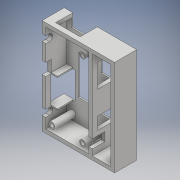
# Autodesk Inventor part: HousingTop
Saved by Autodesk Inventor 2017 (Build 210142000, 142)
## iProperties
Created: 2017-02-14
Part Number: HousingTop
Material: Generic
Document SubType Name: Modeling
Designer: William
Density: 1 g/cm^3
Appearance: Default
Author: William
Autodesk Inventor part; units mm, degrees
ref_plane "YZ Plane" through (0, 0, 0) normal (1, 0, 0) x (0, 1, 0)
ref_plane "XZ Plane" through (0, 0, 0) normal (0, 1, 0) x (-1, 0, 0)
ref_plane "XY Plane" through (0, 0, 0) normal (0, 0, 1) x (1, 0, 0)
sketch "Sketch1" plane through (0, 0, 0) normal (0, 1, 0) x (-1, 0, 0)
  circle A0 centre (0, 0) radius 1.6
  circle A1 centre (0, -62) radius 1.6
  circle A2 centre (25, -62) radius 1.6
  circle A3 centre (12, -31) radius 1.6
  circle A4 centre (12, -31) radius 2.5
  circle A5 centre (0, -62) radius 2.5
  circle A6 centre (25, -62) radius 2.5
  circle A7 centre (0, 0) radius 2.5
  line L0 (30, 5) -> (-5, 5)
  line L1 (-5, 5) -> (-5, -67)
  line L2 (-5, -67) -> (30, -67)
  line L3 (30, -67) -> (30, 5)
  line L4 (33, 8) -> (-8, 8)
  line L5 (-8, 8) -> (-8, -70)
  line L6 (-8, -70) -> (33, -70)
  line L7 (33, -70) -> (33, 8)
  dimension "d0" = 3.2
  dimension "d1" = 3.2
  dimension "d2" = 62
  dimension "d3" = 3.2
  dimension "d4" = 25
  dimension "d5" = 3.2
  dimension "d6" = 31
  dimension "d7" = 12
  dimension "d8" = 5
  dimension "d9" = 5
  dimension "d10" = 5
  dimension "d11" = 5
  dimension "d12" = 5
  dimension "d13" = 5
  dimension "d14" = 5
  dimension "d15" = 5
  dimension "d16" = 3
  dimension "d17" = 3
  dimension "d18" = 3
  dimension "d19" = 3
  dimension "d20" = 0
  constraints: 16 end point, 8 centre point, 5 coincident, 4 parallel, 2 horizontal, 2 perpendicular
  measures "d0" diameter of A0
  measures "d1" diameter of A1
  measures "d2" distance of point (0, 0) A1.centre
  measures "d3" diameter of A2
  measures "d4" distance of A1.centre A2.centre
  measures "d5" diameter of A3
  measures "d6" vertical distance of point (0, 0) A3.centre
  measures "d7" horizontal distance of point (0, 0) A3.centre
  measures "d8" diameter of A4
  measures "d9" diameter of A5
  measures "d10" diameter of A6
  measures "d11" diameter of A7
  measures "d12" distance from line of L2 A2.centre
  measures "d13" distance from line of A2.centre L3
  measures "d14" distance from line of L1 A0.centre
  measures "d15" distance from line of L0 point (0, 0)
  measures "d16" distance between parallel lines of L4 L0
  measures "d17" distance between parallel lines of L3 L7
  measures "d18" distance between parallel lines of L2 L6
  measures "d19" distance between parallel lines of L1 L5
  measures "d20" vertical distance of A1.centre A2.centre
extrude "Extrusion1" add sketch "Sketch1" along normal blind 17 contours A5 | A6 | A7 | L7 L6 L5 L4
sketch "Sketch2" plane through (0, 17, 0) normal (0, 1, 0) x (1, 0, 0)
  line L0 (-33, -8) -> (8, -8) projected
  line L1 (-33, 70) -> (-33, -8) projected
  line L2 (8, -8) -> (-33, -8)
  line L3 (-33, -8) -> (-33, 70)
  line L4 (-33, 70) -> (8, 70)
  line L5 (8, 70) -> (8, -8)
  point P0 (0, 0)
  constraints: 8 end point, 2 parallel, 1 horizontal, 1 perpendicular
extrude "Extrusion2" add sketch "Sketch2" along normal blind 2
sketch "Sketch3" plane through (0, 0, 0) normal (0, -1, 0) x (1, 0, 0)
  line L0 (-33, -70) -> (-33, 8) projected
  line L1 (-30, -67) -> (-30, 5) projected
  line L2 (-33, -30) -> (-30, -30)
  line L3 (-30, -30) -> (-30, -20)
  line L4 (-30, -20) -> (-33, -20)
  line L5 (-33, -20) -> (-33, -30)
  point P0 (0, 0)
  dimension "d25" = 20
  dimension "d26" = 10
  constraints: 8 end point, 2 parallel, 2 point on line, 1 horizontal, 1 perpendicular
  measures "d25" distance from line of point (0, 0) L4
  measures "d26" distance of L4.end L2.start
extrude "Extrusion3" cut sketch "Sketch3" against normal blind 4.5
sketch "Sketch4" plane through (0, 0, 0) normal (0, -1, 0) x (1, 0, 0)
  line L0 (-30, -6.75) -> (-33, -6.75)
  line L1 (-33, -6.75) -> (-33, -1.25)
  line L2 (-33, -1.25) -> (-30, -1.25)
  line L3 (-30, -1.25) -> (-30, -6.75)
  line L4 (-30, -6.75) -> (-33, -1.25) construction
  line L5 (-33, -6.75) -> (-30, -1.25) construction
  line L6 (-30, -20) -> (-30, 5) projected
  line L7 (-33, -20) -> (-33, 8) projected
  line L8 (-30, -58.75) -> (-33, -58.75)
  line L9 (-33, -58.75) -> (-33, -53.25)
  line L10 (-33, -53.25) -> (-30, -53.25)
  line L11 (-30, -53.25) -> (-30, -58.75)
  line L12 (-30, -58.75) -> (-33, -53.25) construction
  line L13 (-33, -58.75) -> (-30, -53.25) construction
  line L14 (-30, -67) -> (-30, -30) projected
  line L15 (-33, -70) -> (-33, -30) projected
  point P0 (0, 0)
  point P1 (-31.5, -4)
  point P2 (-31.5, -56)
  dimension "d29" = 0
  dimension "d30" = 5.5
  dimension "d31" = 0
  dimension "d32" = 4
  dimension "d33" = 0
  dimension "d34" = 0
  dimension "d35" = 56
  dimension "d36" = 5.5
  constraints: 24 end point, 4 midpoint, 4 parallel, 2 horizontal, 2 perpendicular
  measures "d29" distance between parallel lines of L6 L3
  measures "d30" distance of L0.end L1.end
  measures "d31" distance between parallel lines of L7 L1
  measures "d32" vertical distance of point (0, 0) point (-31.5, -4)
  measures "d33" distance between parallel lines of L14 L11
  measures "d34" distance between parallel lines of L15 L9
  measures "d35" vertical distance of point (0, 0) point (-31.5, -56)
  measures "d36" distance between parallel lines of L10 L8
extrude "Extrusion4" cut sketch "Sketch4" against normal blind 5.5
fillet "Fillet1" radius 2.5 4 edges at (-31.5, 5.5, -53.25) (-31.5, 5.5, -58.75) (-31.5, 5.5, -6.75) (-31.5, 5.5, -1.25)
sketch "Sketch5" plane through (0, 17, 0) normal (0, -1, 0) x (1, 0, 0)
  circle A0 centre (0, 0) radius 1.6 projected
  circle A1 centre (0, -62) radius 1.6 projected
  circle A2 centre (-25, -62) radius 1.6 projected
extrude "Extrusion5" cut sketch "Sketch5" against normal up to surface (2 mm away)
sketch "Sketch6" plane through (0, 19, 0) normal (0, 1, 0) x (1, 0, 0)
  line L0 (-23, 42.5) -> (-33, 42.5)
  line L1 (-33, 42.5) -> (-33, 52.5)
  line L2 (-33, 52.5) -> (-23, 52.5)
  line L3 (-23, 52.5) -> (-23, 42.5)
  line L4 (-23, 42.5) -> (-33, 52.5) construction
  line L5 (-33, 42.5) -> (-23, 52.5) construction
  line L6 (-33, -8) -> (-33, 70) projected
  line L7 (-33, 70) -> (8, 70) projected
  line L8 (8, 70) -> (8, -8) projected
  line L9 (8, -8) -> (-33, -8) projected
  circle A0 centre (-25, 62) radius 1.6 projected
  circle A1 centre (0, 62) radius 1.6 projected
  circle A2 centre (0, 0) radius 1.6 projected
  line L10 (-23, 42.5) -> (-33, 42.5)
  line L11 (-33, 42.5) -> (-33, 30.5)
  line L12 (-33, 30.5) -> (-23, 30.5)
  line L13 (-23, 30.5) -> (-23, 42.5)
  point P0 (-28, 47.5)
  dimension "d42" = 47.5
  dimension "d43" = 10
  dimension "d44" = 2
  dimension "d45" = 10
  dimension "d48" = 10
  dimension "d49" = 12
  constraints: 20 end point, 4 parallel, 2 horizontal, 2 midpoint, 2 perpendicular
  measures "d42" vertical distance of point (0, 0) point (-28, 47.5)
  measures "d43" distance of L1.end L2.end
  measures "d44" distance from line of A0.centre L3
  measures "d45" distance of L2.end L0.start
  measures "d48" distance of L12.end L11.end
  measures "d49" distance of L11.end L10.end
extrude "Extrusion6" cut sketch "Sketch6" against normal blind 15 contours L13 L12 L6 L0 | L0 L1 L2 L3
sketch "Sketch7" plane through (0, 17, 0) normal (0, -1, 0) x (1, 0, 0)
  line L0 (-33, -52.5) -> (-30, -52.5) projected
  line L1 (-30, -52.5) -> (-23, -52.5) projected
  line L2 (-23, -52.5) -> (-23, -30.5) projected
  line L3 (-23, -30.5) -> (-30, -30.5) projected
  line L4 (-30, -30.5) -> (-33, -30.5) projected
  line L5 (-33, -30.5) -> (-33, 8) projected
  line L6 (-33, 8) -> (8, 8) projected
  line L7 (8, 8) -> (8, -70) projected
  line L8 (8, -70) -> (-33, -70) projected
  line L9 (-33, -70) -> (-33, -52.5) projected
  line L10 (-30, -52.5) -> (-30, -67) projected
  line L11 (-30, -67) -> (5, -67) projected
  line L12 (5, -67) -> (5, 5) projected
  line L13 (5, 5) -> (-30, 5) projected
  line L14 (-30, 5) -> (-30, -30.5) projected
  circle A0 centre (-25, -62) radius 1.6 projected
  circle A1 centre (-25, -62) radius 2.5 projected
  circle A2 centre (0, -62) radius 1.6 projected
  circle A3 centre (0, -62) radius 2.5 projected
  circle A4 centre (0, 0) radius 1.6 projected
  circle A5 centre (0, 0) radius 2.5 projected
  line L15 (-30, -30.5) -> (-25, -30.5)
  line L16 (-25, -30.5) -> (-25, -29.5)
  line L17 (-25, -29.5) -> (-30, -29.5)
  line L18 (-30, -29.5) -> (-30, -30.5)
  line L19 (-30, -52.5) -> (-25, -52.5)
  line L20 (-25, -52.5) -> (-25, -53.5)
  line L21 (-25, -53.5) -> (-30, -53.5)
  line L22 (-30, -53.5) -> (-30, -52.5)
  dimension "d50" = 5
  dimension "d51" = 1
  dimension "d52" = 5
  dimension "d53" = 1
  constraints: 16 end point, 4 parallel, 2 horizontal, 2 perpendicular
  measures "d50" distance of L17.end L16.end
  measures "d51" distance of L16.end L15.end
  measures "d52" distance of L20.end L21.end
  measures "d53" distance of L19.end L20.end
extrude "Extrusion7" add sketch "Sketch7" along normal up to surface (12.5 mm away) contours L1 L20 L21 L10 | L3 L14 L17 L16
sketch "Sketch8" plane through (0, 19, 0) normal (0, 1, 0) x (1, 0, 0)
  circle A0 centre (0, 0) radius 1.6 construction
  line L0 (0, 0) -> (0, 32.2706) construction
  line L1 (0, 32.2706) -> (-4.4901, 32.2706) construction
  line L2 (-4.4901, 32.2706) -> (-6.7761, 32.2706) construction
  line L3 (-6.7761, 32.2706) -> (-20.4921, 32.2706) construction
  line L4 (-20.4921, 32.2706) -> (-20.4921, 16.2706) construction
  line L5 (-20.4921, 16.2706) -> (-6.7761, 16.2706)
  line L6 (-6.7761, 16.2706) -> (-6.7761, 48.2706)
  line L7 (-6.7761, 48.2706) -> (-20.4921, 48.2706)
  line L8 (-20.4921, 48.2706) -> (-20.4921, 16.2706)
  dimension "d56" = 2.286
  dimension "d57" = 13.716
  dimension "d58" = 16
  dimension "d59" = 32
  constraints: 18 end point, 3 horizontal, 2 parallel, 2 perpendicular, 2 vertical
  measures "d56" distance of L1.end L2.end
  measures "d57" distance of L2.end L3.end
  measures "d58" distance of L3.end L4.end
  measures "d59" distance of L6.end L5.end
extrude "Extrusion8" cut sketch "Sketch8" against normal up to next
sketch "Sketch9" plane through (0, 19, 0) normal (0, 1, 0) x (1, 0, 0)
  line L0 (-33, -8) -> (8, -8) projected
  line L1 (-6, -8) -> (-26, -8)
  line L2 (-26, -8) -> (-26, 2)
  line L3 (-26, 2) -> (-6, 2)
  line L4 (-6, 2) -> (-6, -8)
  line L5 (8, 3) -> (-2, 3)
  line L6 (-2, 3) -> (-2, 22)
  line L7 (-2, 22) -> (8, 22)
  line L8 (8, 22) -> (8, 3)
  line L9 (-2, 41) -> (8, 41)
  line L10 (8, 41) -> (8, 51)
  line L11 (8, 51) -> (-2, 51)
  line L12 (-2, 51) -> (-2, 41)
  line L13 (-2, 41) -> (8, 51) construction
  line L14 (8, 41) -> (-2, 51) construction
  line L15 (8, -8) -> (8, 70) projected
  point P0 (0, 0)
  point P1 (3, 46)
  dimension "d62" = 10
  dimension "d63" = 6
  dimension "d64" = 20
  dimension "d65" = 10
  dimension "d66" = 3
  dimension "d67" = 22
  dimension "d68" = 10
  dimension "d69" = 0
  dimension "d70" = 46
  dimension "d71" = 10
  constraints: 28 end point, 6 parallel, 3 horizontal, 3 perpendicular, 2 midpoint, 1 point on line
  measures "d62" distance of L1.end L2.end
  measures "d63" distance from line of point (0, 0) L4
  measures "d64" distance of L2.end L3.end
  measures "d65" distance of L6.end L7.end
  measures "d66" distance from line of point (0, 0) L5
  measures "d67" vertical distance of point (0, 0) L7.end
  measures "d68" distance between parallel lines of L15 L12
  measures "d69" distance between parallel lines of L15 L10
  measures "d70" vertical distance of point (0, 0) point (3, 46)
  measures "d71" distance of L11.end L9.start
extrude "Extrusion9" cut sketch "Sketch9" against normal blind 15
sketch "Sketch10" plane through (8, 0, 8) normal (1, 0, 0) x (0, 0, -1)
  line L0 (0, 19) -> (11, 19) projected
  line L1 (78, 0) -> (78, 19) projected
  line L2 (0, 19) -> (78, 19)
  line L3 (78, 19) -> (78, 0)
  line L4 (78, 0) -> (0, 0)
  line L5 (0, 0) -> (0, 19)
  point P0 (8, 0)
  constraints: 8 end point, 2 parallel, 1 horizontal, 1 perpendicular
extrude "Extrusion10" add sketch "Sketch10" along normal blind 18
sketch "Sketch11" plane through (0, 0, 0) normal (0, -1, 0) x (1, 0, 0)
  line L0 (23, -67) -> (8, -67)
  line L1 (8, -67) -> (8, 5)
  line L2 (8, 5) -> (23, 5)
  line L3 (23, 5) -> (23, -67)
  line L4 (-33, -70) -> (26, -70) projected
  line L5 (26, 8) -> (26, -70) projected
  line L6 (5, -67) -> (5, -51) projected
  line L7 (-33, 8) -> (26, 8) projected
  point P0 (0, 0)
  dimension "d76" = 3
  dimension "d77" = 3
  dimension "d78" = 3
  dimension "d79" = 3
  constraints: 8 end point, 2 parallel, 1 horizontal, 1 perpendicular
  measures "d76" distance between parallel lines of L4 L0
  measures "d77" distance between parallel lines of L5 L3
  measures "d78" distance between parallel lines of L6 L1
  measures "d79" distance between parallel lines of L7 L2
extrude "Extrusion11" cut sketch "Sketch11" against normal up to surface (17 mm away)
sketch "Sketch12" plane through (0, 0, 0) normal (0, -1, 0) x (1, 0, 0)
  line L0 (8, -51) -> (8, -67) projected
  line L1 (5, 5) -> (5, -67) projected
  line L2 (8, -54.794) -> (5, -54.794)
  line L3 (5, -54.794) -> (5, -62.0092)
  line L4 (5, -62.0092) -> (8, -62.0092)
  line L5 (8, -62.0092) -> (8, -54.794)
  point P0 (0, 0)
  constraints: 8 end point, 2 parallel, 2 point on line, 1 horizontal, 1 perpendicular
extrude "Extrusion12" cut sketch "Sketch12" against normal blind 10
chamfer "Chamfer1" distance 1 angle 45 24 edges at (-3.5, 19, -70) (26, 19, -31) (-33, 19, -61.25) (-28, 19, -52.5) (-23, 19, -41.5) (-28, 19, -30.5) (-33, 19, -11.25) (-20.4921, 19, -32.2706) (-13.6341, 19, -48.2706) (-6.7761, 19, -32.2706) (-13.6341, 19, -16.2706) (3, 19, -3) (8, 19, -12.5) (3, 19, -22) (-2, 19, -12.5) (3, 19, -41) (8, 19, -46) (3, 19, -51) (-2, 19, -46) (-6, 19, 3) (-16, 19, -2) (-29.5, 19, 8) (-26, 19, 3) (10, 19, 8)
body "Solid1"
